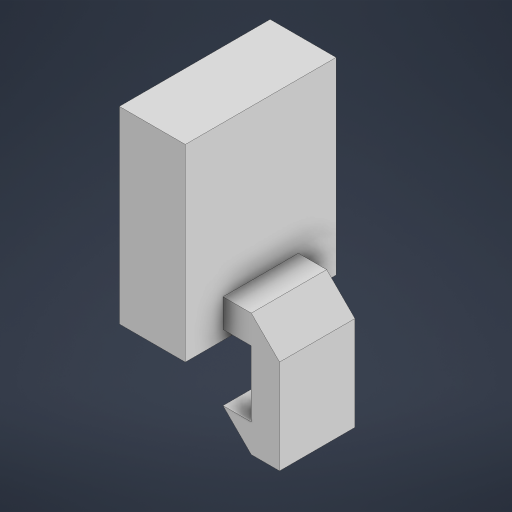
# Autodesk Inventor part: prueba_up
Saved by Autodesk Inventor 2024.1 (Build 281209000, 209)
## iProperties
Created: 2023-07-21
Part Number: prueba_up
Material: Generic
Document SubType Name: Modeling
Designer: LabTel_Admin
Density: 1 g/cm^3
Appearance: Default
Author: LabTel_Admin
Autodesk Inventor part; units mm, degrees
ref_plane "YZ Plane" through (0, 0, 0) normal (1, 0, 0) x (0, 1, 0)
ref_plane "XZ Plane" through (0, 0, 0) normal (0, 1, 0) x (-1, 0, 0)
ref_plane "XY Plane" through (0, 0, 0) normal (0, 0, 1) x (1, 0, 0)
sketch "Sketch1" plane through (0, 0, 0) normal (0, 1, 0) x (-1, 0, 0)
  line L0 (-1.75, -4) -> (1.75, -4)
  line L1 (1.75, -4) -> (1.75, 4)
  line L2 (1.75, 4) -> (-1.75, 4)
  line L3 (-1.75, 4) -> (-1.75, -4)
  line L4 (-1.75, -4) -> (1.75, 4) construction
  line L5 (1.75, -4) -> (-1.75, 4) construction
  point P0 (0, 0)
  dimension "d0" = 3.5
  dimension "d1" = 8
  constraints: 12 end point, 2 midpoint, 2 parallel, 1 horizontal, 1 perpendicular
  measures "d0" distance of L2.end L1.end
  measures "d1" distance of L0.end L1.end
extrude "Extrusion1" add sketch "Sketch1" along normal blind 10
sketch "Sketch2" plane through (1.75, 0, 4) normal (1, 0, 0) x (0, 0, -1)
  line L0 (2, 2) -> (6, 2)
  line L1 (6, 2) -> (6, 0.5)
  line L2 (6, 0.5) -> (2, 0.5)
  line L3 (2, 0.5) -> (2, 2)
  line L4 (8, 0) -> (8, 10) projected
  line L5 (0, 0) -> (8, 0) projected
  point P0 (4, 0)
  dimension "d4" = 2
  dimension "d5" = 4
  dimension "d6" = 1.5
  dimension "d7" = 0.5
  constraints: 8 end point, 2 parallel, 1 horizontal, 1 perpendicular
  measures "d4" distance between parallel lines of L4 L1
  measures "d5" distance of L1.end L2.end
  measures "d6" distance of L2.end L0.start
  measures "d7" distance between parallel lines of L5 L2
extrude "Extrusion2" add sketch "Sketch2" along normal blind 3
sketch "Sketch3" plane through (1.75, 0.5, -2) normal (0, -1, 0) x (1, 0, 0)
  line L0 (3, 0) -> (3, 4) projected
  line L1 (0, 0) -> (3, 0) projected
  line L2 (3, 4) -> (1.5, 4)
  line L3 (1.5, 4) -> (1.5, 0)
  line L4 (1.5, 0) -> (3, 0)
  line L5 (3, 0) -> (3, 4)
  point P0 (-1.75, 2)
  constraints: 8 end point, 2 parallel, 1 horizontal, 1 midpoint, 1 perpendicular
extrude "Extrusion3" add sketch "Sketch3" along normal blind 5
sketch "Sketch4" plane through (3.25, 0.5, -2) normal (-1, 0, 0) x (0, 0, 1)
  line L0 (4, 1.5) -> (4, -5) projected
  line L1 (4, -5) -> (-0.0639, -5)
  line L2 (-0.0639, -5) -> (-0.0639, -3.5)
  line L3 (-0.0639, -3.5) -> (4, -3.5)
  line L4 (4, -3.5) -> (4, -5)
  point P0 (2, -0.5)
  dimension "d12" = 1.5
  constraints: 8 end point, 2 parallel, 1 horizontal, 1 perpendicular
  measures "d12" distance of L1.end L2.end
extrude "Extrusion4" add sketch "Sketch4" along normal blind 1.5
sketch "Sketch5" plane through (1.75, 0.5, 2) normal (0, 0, 1) x (1, 0, 0)
  line L0 (1.5, -3.5) -> (0, -3.5) projected
  line L1 (3, -5) -> (0, -5) projected
  line L2 (0, 1.5) -> (3, 1.5) projected
  line L3 (1.5, 1.5) -> (3, 0)
  line L4 (3, 1.5) -> (3, -5) projected
  line L5 (1.5, -3.5) -> (1.5, -5) projected
  line L6 (1.5, -5) -> (0, -3.5)
  line L7 (3, 0) -> (3, 1.5)
  line L8 (3, 1.5) -> (1.5, 1.5)
  line L9 (1.5, -5) -> (0, -5)
  line L10 (0, -5) -> (0, -3.5) projected
  line L11 (0, -3.5) -> (0, -5)
  point P0 (-1.75, -0.5)
  dimension "d15" = 1.5
  dimension "d16" = 1.5
  constraints: 12 end point, 2 collinear, 1 midpoint, 1 perpendicular, 1 point on line, 1 vertical
  measures "d15" distance of L2.end L3.end
  measures "d16" distance of L2.end L3.start
extrude "Extrusion5" cut sketch "Sketch5" against normal through all contours L6 L1 L10 | L2 L4 L3
body "Solid1"
